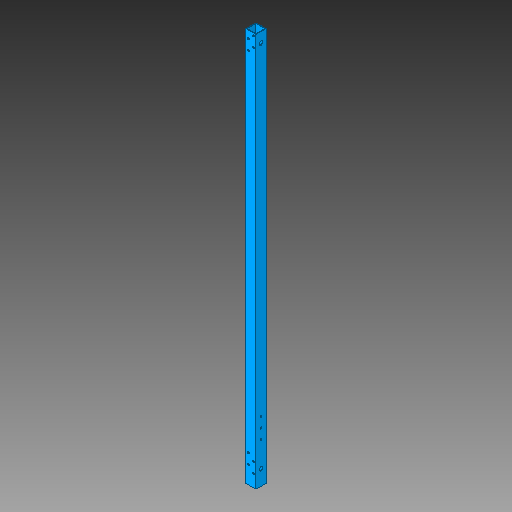
# Autodesk Inventor part: ElvFrontBeam
Saved by Autodesk Inventor 2019 (Build 230136000, 136)
## iProperties
Created: 2019-01-09
Part Number: ElvFrontBeam
Material: Aluminum 6061
Document SubType Name: Modeling
Designer: james
Density: 2.7 g/cm^3
Appearance: Default(3)
Mass: 404.212 g
Surface Area: 1889.91 cm^2
Volume: 149.708 cm^3
Author: james
Autodesk Inventor part; units mm, degrees
ref_plane "YZ Plane" through (0, 0, 0) normal (1, 0, 0) x (0, 1, 0)
ref_plane "XZ Plane" through (0, 0, 0) normal (0, 1, 0) x (-1, 0, 0)
ref_plane "XY Plane" through (0, 0, 0) normal (0, 0, 1) x (1, 0, 0)
sketch "Sketch1" plane through (0, 0, 0) normal (0, 1, 0) x (-1, 0, 0)
  line L0 (17.0295, 14.999) -> (-8.3705, 14.999)
  line L1 (-8.3705, 14.999) -> (-8.3705, -10.401)
  line L2 (-8.3705, -10.401) -> (17.0295, -10.401)
  line L3 (17.0295, -10.401) -> (17.0295, 14.999)
  line L4 (15.442, -8.8135) -> (-6.783, -8.8135)
  line L5 (-6.783, -8.8135) -> (-6.783, 13.4115)
  line L6 (-6.783, 13.4115) -> (15.442, 13.4115)
  line L7 (15.442, 13.4115) -> (15.442, -8.8135)
  point P0 (0, 0)
  dimension "d0" = 25.4
  dimension "d1" = 25.4
  dimension "d4" = 1.5875
  dimension "d5" = 1.5875
  dimension "d6" = 1.5875
  dimension "d7" = 1.5875
  constraints: 16 end point, 4 parallel, 2 horizontal, 2 perpendicular
  measures "d0" distance of L0.end L1.end
  measures "d1" distance of L0.start L0.end
  measures "d4" distance between parallel lines of L0 L6
  measures "d5" distance between parallel lines of L2 L4
  measures "d6" distance between parallel lines of L3 L7
  measures "d7" distance between parallel lines of L1 L5
extrude "Extrusion2" add sketch "Sketch1" along normal blind 990.6
sketch "Sketch6" plane through (8.3705, 0, 14.999) normal (1, 0, 0) x (0, 0, -1)
  line L0 (25.4, 0) -> (25.4, 990.6) projected
  line L1 (0, 0) -> (25.4, 0) projected
  point P0 (14.999, 0)
  point P1 (12.7, 38.1)
  dimension "d46" = 12.7
  dimension "d47" = 38.1
  measures "d46" distance from line of point (12.7, 38.1) L0
  measures "d47" distance from line of L1 point (12.7, 38.1)
hole "Hole5" at (8.3705, 38.1, 2.299) direction (-1, 0, 0) diameter 9.5758 depth 25.4 tip angle 118
sketch "Sketch7" plane through (8.3705, 0, 14.999) normal (1, 0, 0) x (0, 0, -1)
  line L0 (25.4, 0) -> (25.4, 990.6) projected
  line L1 (0, 990.6) -> (25.4, 990.6) projected
  point P0 (14.999, 0)
  point P1 (12.7, 965.2)
  dimension "d55" = 12.7
  dimension "d56" = 25.4
  measures "d55" distance from line of L0 point (12.7, 965.2)
  measures "d56" distance from line of L1 point (12.7, 965.2)
hole "Hole6" at (8.3705, 965.2, 2.299) direction (-1, 0, 0) diameter 9.5758 depth 25.4 tip angle 118
sketch "Sketch8" plane through (8.3705, 0, 14.999) normal (1, 0, 0) x (0, 0, -1)
  line L0 (0, 0) -> (25.4, 0) projected
  line L1 (25.4, 0) -> (25.4, 990.6) projected
  point P0 (14.999, 0)
  point P1 (12.7, 101.6)
  point P2 (12.7, 127)
  point P3 (12.7, 152.4)
  dimension "d64" = 25.4
  dimension "d65" = 25.4
  dimension "d66" = 101.6
  dimension "d67" = 12.7
  dimension "d68" = 0
  dimension "d69" = 0
  measures "d64" distance of point (12.7, 127) point (12.7, 152.4)
  measures "d65" distance of point (12.7, 101.6) point (12.7, 127)
  measures "d66" distance from line of L0 point (12.7, 101.6)
  measures "d67" distance from line of L1 point (12.7, 101.6)
  measures "d68" horizontal distance of point (12.7, 101.6) point (12.7, 127)
  measures "d69" horizontal distance of point (12.7, 127) point (12.7, 152.4)
hole "Hole7" at (8.3705, 101.6, 2.299) at (8.3705, 127, 2.299) at (8.3705, 152.4, 2.299) direction (-1, 0, 0) diameter 4.826 depth 25.4 tip angle 118
sketch "Sketch9" plane through (-17.0295, 0, 14.999) normal (0, 0, 1) x (1, 0, 0)
  line L0 (25.4, 0) -> (25.4, 990.6) projected
  line L1 (0, 990.6) -> (25.4, 990.6) projected
  line L2 (0, 0) -> (0, 990.6) projected
  point P0 (17.0295, 0)
  point P1 (19.05, 984.25)
  point P2 (6.35, 971.55)
  point P3 (19.05, 958.85)
  point P4 (6.35, 946.15)
  dimension "d77" = 6.35
  dimension "d78" = 6.35
  dimension "d79" = 6.35
  dimension "d80" = 6.35
  dimension "d81" = 6.35
  dimension "d82" = 19.05
  dimension "d83" = 25.4
  dimension "d84" = 25.4
  measures "d77" distance from line of L0 point (19.05, 984.25)
  measures "d78" distance from line of L1 point (19.05, 984.25)
  measures "d79" distance from line of L2 point (6.35, 971.55)
  measures "d80" distance from line of L2 point (6.35, 946.15)
  measures "d81" distance from line of L0 point (19.05, 958.85)
  measures "d82" distance from line of L1 point (6.35, 971.55)
  measures "d83" distance of point (6.35, 946.15) point (6.35, 971.55)
  measures "d84" distance of point (19.05, 958.85) point (19.05, 984.25)
hole "Hole8" at (2.0205, 984.25, 14.999) at (-10.6795, 971.55, 14.999) at (2.0205, 958.85, 14.999) at (-10.6795, 946.15, 14.999) direction (0, 0, -1) diameter 4.7625 depth 25.4 tip angle 118
sketch "Sketch10" plane through (-17.0295, 0, 14.999) normal (0, 0, 1) x (1, 0, 0)
  line L0 (25.4, 0) -> (25.4, 990.6) projected
  line L1 (0, 0) -> (0, 990.6) projected
  line L2 (0, 0) -> (25.4, 0) projected
  point P0 (17.0295, 0)
  point P1 (6.35, 69.85)
  point P2 (19.05, 57.15)
  point P3 (6.35, 44.45)
  point P4 (19.05, 31.75)
  dimension "d92" = 6.35
  dimension "d93" = 6.35
  dimension "d94" = 6.35
  dimension "d95" = 6.35
  dimension "d96" = 25.4
  dimension "d97" = 25.4
  dimension "d98" = 31.75
  dimension "d99" = 44.45
  measures "d92" distance from line of L0 point (19.05, 57.15)
  measures "d93" distance from line of L0 point (19.05, 31.75)
  measures "d94" distance from line of L1 point (6.35, 44.45)
  measures "d95" distance from line of L1 point (6.35, 69.85)
  measures "d96" distance of point (19.05, 31.75) point (19.05, 57.15)
  measures "d97" distance of point (6.35, 69.85) point (6.35, 44.45)
  measures "d98" distance from line of point (19.05, 31.75) L2
  measures "d99" distance from line of L2 point (6.35, 44.45)
hole "Hole9" at (-10.6795, 69.85, 14.999) at (2.0205, 57.15, 14.999) at (-10.6795, 44.45, 14.999) at (2.0205, 31.75, 14.999) direction (0, 0, -1) diameter 4.7625 depth 25.4 tip angle 118
equation "\"d0\" = ElvBeamWidth"
equation "\"d1\" = ElvBeamWidth"
equation "\"d4\" = ElvWallWidth"
equation "\"d5\" = ElvWallWidth"
equation "\"d6\" = ElvWallWidth"
equation "\"d7\" = ElvWallWidth"
equation "\"d8\" = ElvFrontBeamLength"
equation "\"d47\" = ElvHoleFromBottom"
equation "\"d56\" = ElvHoleFromFront"
equation "\"ElvMiddleBeamLength\" = 990.6"
equation "\"ElvWallWidth\" = 1.5875"
equation "\"ElvFrontBeamLength\" = 990.6"
equation "\"ElvEndEffectLength\" = 406.4"
equation "\"ElvCrossBeamLength\" = 304.8"
equation "\"ElvBeamWidth\" = 25.4"
equation "\"ElvFrontBeamLength_1\" = 1066.8"
equation "\"ElvFixedBeamLength\" = 990.6"
equation "\"ElvDelFrontTabLength\" = 6.35"
equation "\"ElvDelDepth\" = 6.35"
equation "\"ElvDelHeight\" = 101.6"
equation "\"ElvDelWidth\" = 18.542"
equation "\"ElvTopBeamLength\" = 457.2"
equation "\"ElvHoleFromBottom\" = 38.1"
equation "\"ElvHoleFromMid\" = 38.1"
equation "\"ElvHoleFromFixed\" = 50.8"
equation "\"ElvHoleFromFront\" = 25.4"
equation "\"ElvRivetPlateLength\" = 76.2"
equation "\"ElvDelMiddleTabLength\" = 6.35"
body "Solid2"
